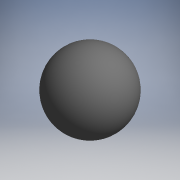
# Autodesk Inventor part: F624ZZ Ball
Saved by Autodesk Inventor 2017.3 (Build 213256000, 256)
## iProperties
Part Number: F624ZZ Ball
Material: Generic
Catalog Web Link: www.cadenas.de
Description: shielded_type_zz_zzs_B-
Vendor: NSK_RB
Document SubType Name: Modeling
Designer: partserver
Manufacturer: NSK_RB
Mass: 0.010306 g
Surface Area: 0.229022 cm^2
Volume: 0.010306 cm^3
Density: 1 g/cm^3
Appearance: PSOLRGB-128-128-128
Category: PARTsolutions
Company: NSK_RB
Title: F624ZZ Ball
Author: Cadenas PARTsolutions
PSOL_IDENT_0: {$CADENAS_DATA\23d-libs\nsk_rb\roller_bearings\deep_groove_bb\exstra_small_miniatur_bb\metric_design
PSOL_IDENT_1: _with_flange\shielded_type_zz_zzs_b_1.prj},179 {VTYP=3D},{NB=F624ZZ Ball},{LINA=F624ZZ Ball},{NN=shi
PSOL_IDENT_2: elded_type_zz_zzs_B},{DATE=16.07.2021 00:25:32},{GEOMDATE=04.01.2008 00:00:00},{VERSION=},{LINEID=23
PSOL_IDENT_3: 0},{WBVAR=},{WBNUMERIC=}  {NB=F624ZZ Ball},{LINA=F624ZZ Ball},{KT=DUMMY},{IDNR=},{STAN=},{ORDER=F624
PSOL_IDENT_4: ZZ},{SD=4.0},{X=4.0},{D=13},{DD=13},{DD1=0.0},{D2=15.0},{DD2=15.0},{B=0.0},{B1=5.0},{CC1=0.0},{C2=1.
PSOL_IDENT_5: 0},{CC2=1.0},{R=0.00},{R1=0.20},{DI1=6.95},{DI2=6.00},{SDE1=10.45},{SDE2=11.30},{CR1=1300},{COR1=485
PSOL_IDENT_6: },{CR2=133},{COR2=49.0},{LG=40000},{LO=48000},{DA=0.0},{DB=6.0},{RA=0.00},{RB=0.20},{MASS=3.53},{SC=
PSOL_IDENT_7: 1}
NB: F624ZZ Ball
NN: shielded_type_zz_zzs_B
NBSYN: $ORDER. Ball
LINA: F624ZZ Ball
CATALOG: NSK Rolling Bearing
ORDER: F624ZZ
SD: 4
X: 4
D: 13
DD: 13
DD1: 0
D2: 15
DD2: 15
B: 0
B1: 5
CC1: 0
C2: 1
CC2: 1
R: 0
R1: 0.2
DI1: 6.95
DI2: 6
SDE1: 10.45
SDE2: 11.3
CR1: 1300
COR1: 485
CR2: 133
COR2: 49
LG: 40000
LO: 48000
DA: 0
DB: 6
RA: 0
RB: 0.2
MASS: 3.53
SC: 1
SUPPLIER: NSK_RB
ARTICLENO: F624ZZ Ball
BOMINFO: F624ZZ Ball
CREATOR: CADENAS GmbH
Autodesk Inventor part; units mm, degrees
sketch "Sketch_1" plane through (0, 0, 0) normal (0, 0, 1) x (1, 0, 0)
  line L0 (1.35, 0) -> (-1.35, 0)
  arc A0 (1.35, 0) -> (-1.35, 0) centre (0, 0) ccw
  line L1 (1.35, 0) -> (-1.35, 0)
  constraints: 4 end point, 2 point on circle, 1 centre point
revolve "Revolution1" add sketch "Sketch_1" angle 360 about axis through (1.35, 0, 0) along (1, 0, 0)
ref_plane "ip_st_1_XY" through (0, 0, 0) normal (-1, 0, 0) x (0, 0, -1)
ref_plane "ip_st_1_YZ" through (0, 0, 0) normal (0, 0, -1) x (0, -1, 0)
ref_plane "ip_st_1_ZX" through (0, 0, 0) normal (0, -1, 0) x (-1, 0, 0)
body "Solid1"
